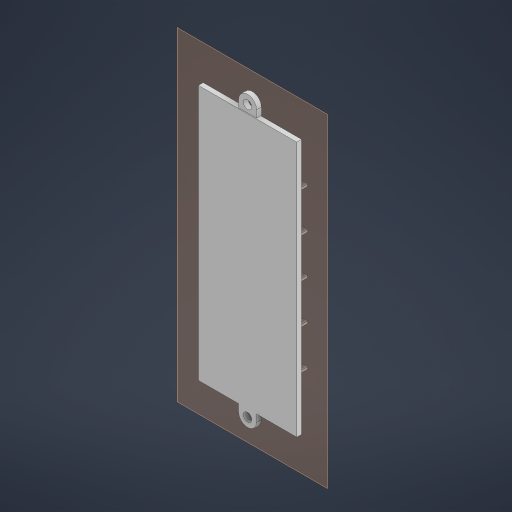
# Autodesk Inventor part: light fixture
Saved by Autodesk Inventor 2024.3 (Build 283343000, 343)
## iProperties
Created: 2025-08-06
Part Number: light fixture
Material: Generic
Document SubType Name: Modeling
Designer: giuseppe
Density: 1 g/cm^3
Appearance: Default
Author: giuseppe
## iProperties of the stored document light fixture_3DPrint.ipt
Created: 2025-08-08
Part Number: light fixture_3DPrint
Material: Generic
Document SubType Name: Modeling
Designer: giuseppe
Density: 1 g/cm^3
Appearance: Default
Author: giuseppe
Autodesk Inventor part; units mm, degrees
ref_plane "YZ Plane" through (0, 0, 0) normal (1, 0, 0) x (0, 1, 0)
ref_plane "XZ Plane" through (0, 0, 0) normal (0, 1, 0) x (-1, 0, 0)
ref_plane "XY Plane" through (0, 0, 0) normal (0, 0, 1) x (1, 0, 0)
ref_plane "Work Plane1" through (0, 0, 6) normal (0, 0, 1) x (1, 0, 0)
sketch "Sketch1" plane through (0, 0, 6) normal (0, 0, 1) x (1, 0, 0)
  line L0 (20.5, 53.1) -> (-20.5, 53.1) projected
  line L1 (-20.5, 53.1) -> (-20.5, -53.4) projected
  line L2 (-20.5, -53.4) -> (20.5, -53.4) projected
  line L3 (20.5, -53.4) -> (20.5, 53.1) projected
  line L4 (-18.5, 51.4) -> (-18.5, -51.4) projected
  line L5 (18.5, 51.4) -> (-18.5, 51.4) projected
  line L6 (18.5, -51.4) -> (18.5, 51.4) projected
  line L7 (-18.5, -51.4) -> (18.5, -51.4) projected
  point P0 (0, 0)
extrude "Extrusion1" add sketch "Sketch1" along normal blind 2 contours L3 L2 L1 L0 | L5 L6 L7 L4
sketch "Sketch2" plane through (0, 0, 8) normal (0, 0, 1) x (1, 0, 0)
  line L0 (-3.75, -53.4) -> (3.75, -53.4)
  line L1 (3.75, -53.4) -> (3.75, -56.4)
  line L2 (3.75, -56.4) -> (-3.75, -56.4)
  line L3 (-3.75, -56.4) -> (-3.75, -53.4)
  arc A0 (-3.75, -56.4) -> (3.75, -56.4) centre (0, -56.4) ccw
  circle A1 centre (0, -56.4) radius 1.75
  line L4 (-20.5, -53.4) -> (20.5, -53.4) projected
  point P0 (0, 0)
  dimension "d2" = 3.5
  dimension "d3" = 2
  dimension "d4" = 3
  constraints: 8 end point, 2 centre point, 2 parallel, 2 point on circle, 1 coincident, 1 collinear, 1 horizontal, 1 midpoint, 1 perpendicular, 1 vertical alignment
  measures "d2" diameter of A1
  measures "d3" radial gap between concentric circles of A0 A1
  measures "d4" distance of L2.end L0.start
extrude "Extrusion2" add sketch "Sketch2" against normal up to surface (2 mm away) contours L0 L1 L2 A1 L3 | L2 A1 A0
mirror "Mirror1" about plane through (0, 0, 0) normal (0, 1, 0) of "Extrusion2"
sketch "Sketch3" plane through (0, 0, 6) normal (0, 0, -1) x (-1, 0, 0)
  line L0 (2, -8.7527) -> (2, -14.9) projected
  line L1 (2, -14.9) -> (-17, -5.4024) projected
  line L2 (-17, -5.4024) -> (-2, -8.0473) projected
  line L3 (-2, -8.0473) -> (-2, -1.9) projected
  line L4 (-2, -1.9) -> (17, -11.3976) projected
  line L5 (17, -11.3976) -> (2, -8.7527) projected
  line L6 (2, 40.7473) -> (2, 34.6) projected
  line L7 (2, 34.6) -> (-17, 44.0976) projected
  line L8 (-17, 44.0976) -> (-2, 41.4527) projected
  line L9 (-2, 41.4527) -> (-2, 47.6) projected
  line L10 (-2, 47.6) -> (17, 38.1024) projected
  line L11 (17, 38.1024) -> (2, 40.7473) projected
  line L12 (2, -25.2527) -> (2, -31.4) projected
  line L13 (2, -31.4) -> (-17, -21.9024) projected
  line L14 (-17, -21.9024) -> (-2, -24.5473) projected
  line L15 (-2, -24.5473) -> (-2, -18.4) projected
  line L16 (-2, -18.4) -> (17, -27.8976) projected
  line L17 (17, -27.8976) -> (2, -25.2527) projected
  line L18 (2, 7.7473) -> (2, 1.6) projected
  line L19 (2, 1.6) -> (-17, 11.0976) projected
  line L20 (-17, 11.0976) -> (-2, 8.4527) projected
  line L21 (-2, 8.4527) -> (-2, 14.6) projected
  line L22 (-2, 14.6) -> (17, 5.1024) projected
  line L23 (17, 5.1024) -> (2, 7.7473) projected
  line L24 (2, 24.2473) -> (2, 18.1) projected
  line L25 (2, 18.1) -> (-17, 27.5976) projected
  line L26 (-17, 27.5976) -> (-2, 24.9527) projected
  line L27 (-2, 24.9527) -> (-2, 31.1) projected
  line L28 (-2, 31.1) -> (17, 21.6024) projected
  line L29 (17, 21.6024) -> (2, 24.2473) projected
  line L30 (2, -41.7527) -> (2, -47.9) projected
  line L31 (2, -47.9) -> (-17, -38.4024) projected
  line L32 (-17, -38.4024) -> (-2, -41.0473) projected
  line L33 (-2, -41.0473) -> (-2, -34.9) projected
  line L34 (-2, -34.9) -> (17, -44.3976) projected
  line L35 (17, -44.3976) -> (2, -41.7527) projected
  line L36 (-20, 52.6) -> (-20, -52.9) projected
  line L37 (-20, -52.9) -> (20, -52.9) projected
  line L38 (20, -52.9) -> (20, 52.6) projected
  line L39 (20, 52.6) -> (-20, 52.6) projected
  line L40 (-18, -33.6) -> (17.5, -33.6)
  line L41 (17.5, -33.6) -> (17.5, -32.7)
  line L42 (17.5, -32.7) -> (-18, -32.7)
  line L43 (-18, -32.7) -> (-18, -33.6)
  line L44 (20.5, 53.1) -> (20.5, -53.4) projected
  point P0 (0, 0)
  point P1 (-18, -33.15)
  dimension "d7" = 1.3
  dimension "d8" = 1.3
  dimension "d9" = 2
  dimension "d10" = 3
  constraints: 8 end point, 2 parallel, 1 horizontal, 1 midpoint, 1 perpendicular
  measures "d7" distance from line of L40 L33.end
  measures "d8" distance from line of L42 L12.end
  measures "d9" distance from line of L36 point (-18, -33.15)
  measures "d10" distance between parallel lines of L44 L41
extrude "Extrusion3" add sketch "Sketch3" along normal blind 5 contours L43 L42 L41 L40
pattern_linear "Rectangular Pattern1" count 5 spacing 16.5 along (0, 1, 0) of "Extrusion3"
body "Solid1"
